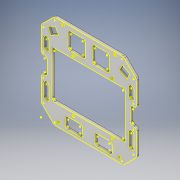
# Autodesk Inventor part: AnilloBaseVTOLv2
Saved by Autodesk Inventor 2019 (Build 230136000, 136)
## iProperties
Created: 2019-02-06
Part Number: AnilloBaseVTOLv2
Material: Generic
Document SubType Name: Modeling
Designer: Kenny
Density: 1 g/cm^3
Appearance: Default
Author: Kenny
Autodesk Inventor part; units mm, degrees
ref_plane "YZ Plane" through (0, 0, 0) normal (1, 0, 0) x (0, 1, 0)
ref_plane "XZ Plane" through (0, 0, 0) normal (0, 1, 0) x (-1, 0, 0)
ref_plane "XY Plane" through (0, 0, 0) normal (0, 0, 1) x (1, 0, 0)
sketch "Sketch1" plane through (0, 0, 0) normal (0, 0, 1) x (1, 0, 0)
  line L0 (0, 0) -> (110, 0)
  line L1 (110, 108) -> (0, 108)
  line L2 (55, 108) -> (55, 0) construction
  line L3 (12.5, 77) -> (97.5, 77)
  line L4 (97.5, 77) -> (97.5, 23)
  line L5 (97.5, 23) -> (12.5, 23)
  line L6 (12.5, 23) -> (12.5, 77)
  line L7 (-68.3542, 85.0055) -> (-13.3542, 85.0055) construction
  line L8 (-13.3542, 85.0055) -> (-13.3542, 15.0055) construction
  line L9 (-13.3542, 15.0055) -> (-68.3542, 15.0055) construction
  line L10 (-68.3542, 15.0055) -> (-68.3542, 85.0055) construction
  line L11 (49.5525, 105.4569) -> (59.7609, 105.4569) construction
  line L12 (59.7609, 105.4569) -> (59.7609, 101.2404) construction
  line L13 (59.7609, 101.2404) -> (49.5525, 101.2404) construction
  line L14 (49.5525, 101.2404) -> (49.5525, 105.4569) construction
  line L15 (0, 64) -> (7, 64)
  line L16 (7, 64) -> (7, 44)
  line L17 (7, 44) -> (0, 44)
  line L18 (0, 108) -> (0, 64)
  line L19 (0, 44) -> (0, 0)
  line L20 (110, 0) -> (110, 44)
  line L21 (110, 64) -> (110, 108)
  line L22 (59, 103) -> (79, 103)
  line L23 (79, 103) -> (79, 83)
  line L24 (79, 83) -> (59, 83)
  line L25 (59, 83) -> (59, 103)
  line L26 (31, 103) -> (51, 103)
  line L27 (51, 103) -> (51, 83)
  line L28 (51, 83) -> (31, 83)
  line L29 (31, 83) -> (31, 103)
  line L30 (3, 84) -> (9, 84)
  line L31 (9, 84) -> (9, 69)
  line L32 (9, 69) -> (3, 69)
  line L33 (3, 69) -> (3, 84)
  line L34 (101, 84) -> (107, 84)
  line L35 (107, 84) -> (107, 69)
  line L36 (107, 69) -> (101, 69)
  line L37 (101, 69) -> (101, 84)
  line L38 (62, 16) -> (82, 16)
  line L39 (82, 16) -> (82, 3)
  line L40 (82, 3) -> (62, 3)
  line L41 (62, 3) -> (62, 16)
  line L42 (28, 16) -> (48, 16)
  line L43 (48, 16) -> (48, 3)
  line L44 (48, 3) -> (28, 3)
  line L45 (28, 3) -> (28, 16)
  line L46 (110, 108) -> (110, 0) construction
  line L47 (110, 64) -> (103, 64)
  line L48 (103, 64) -> (103, 44)
  line L49 (103, 44) -> (110, 44)
  line L50 (9, 39) -> (3, 39)
  line L51 (3, 39) -> (3, 19)
  line L52 (3, 19) -> (9, 19)
  line L53 (9, 19) -> (9, 39)
  line L54 (101, 39) -> (107, 39)
  line L55 (107, 39) -> (107, 19)
  line L56 (107, 19) -> (101, 19)
  line L57 (101, 19) -> (101, 39)
  line L58 (0, 108) -> (20, 108)
  line L59 (20, 108) -> (20, 92) construction
  line L60 (20, 92) -> (0, 92) construction
  line L61 (0, 92) -> (0, 108)
  line L62 (110, 108) -> (90, 108)
  line L63 (90, 108) -> (90, 92) construction
  line L64 (90, 92) -> (110, 92) construction
  line L65 (110, 92) -> (110, 108)
  line L66 (90, 92) -> (98.9879, 87.6163)
  line L67 (98.9879, 87.6163) -> (102.4949, 94.8066)
  line L68 (102.4949, 94.8066) -> (93.507, 99.1904)
  line L69 (93.507, 99.1904) -> (90, 92)
  line L70 (20, 92) -> (11.0121, 87.6163)
  line L71 (11.0121, 87.6163) -> (7.5051, 94.8066)
  line L72 (7.5051, 94.8066) -> (16.493, 99.1904)
  line L73 (16.493, 99.1904) -> (20, 92)
  point P0 (25, 105)
  point P1 (85, 105)
  point P2 (20, 5)
  point P3 (90, 5)
  point P4 (-63.3542, 80.0055)
  point P5 (-63.3542, 20.0055)
  point P6 (-18.3542, 80.0055)
  point P7 (-18.3542, 20.0055)
  point P8 (37, 20)
  point P9 (82, 20)
  point P10 (37, 80)
  point P11 (82, 80)
  point P12 (104, 84)
  point P13 (6, 84)
  point P14 (41, 83)
  point P15 (72, 16)
  point P16 (6, 39)
  point P17 (104, 39)
  point P18 (41, 103)
  point P19 (69, 103)
  dimension "d0" = 60
  dimension "d1" = 100
  dimension "d2" = 70
  dimension "d3" = 110
  dimension "d4" = 108
  dimension "d6" = 35
  dimension "d7" = 5
  dimension "d8" = 85
  dimension "d9" = 54
  dimension "d11" = 45
  dimension "d12" = 60
  dimension "d14" = 23
  dimension "d15" = 55
  dimension "d16" = 70
  dimension "d17" = 5
  dimension "d18" = 5
  dimension "d23" = 28
  dimension "d24" = 20
  dimension "d29" = 7
  dimension "d30" = 20
  dimension "d35" = 12.5
  dimension "d36" = 12.5
  dimension "d38" = 20
  dimension "d39" = 20
  dimension "d40" = 25
  dimension "d41" = 45
  dimension "d42" = 28
  dimension "d43" = 20
  dimension "d44" = 20
  dimension "d46" = 31
  dimension "d47" = 6
  dimension "d48" = 15
  dimension "d49" = 6
  dimension "d50" = 15
  dimension "d51" = 3
  dimension "d52" = 3
  dimension "d53" = 31
  dimension "d54" = 20
  dimension "d55" = 13
  dimension "d56" = 20
  dimension "d57" = 13
  dimension "d58" = 28
  dimension "d59" = 28
  dimension "d60" = 7
  dimension "d62" = 7
  dimension "d63" = 20
  dimension "d64" = 6
  dimension "d65" = 20
  dimension "d66" = 6
  dimension "d67" = 20
  dimension "d68" = 3
  dimension "d69" = 3
  dimension "d70" = 5
  dimension "d71" = 5
  dimension "d72" = 5
  dimension "d73" = 7
  dimension "d74" = 19
  dimension "d75" = 5
  dimension "d137" = 20
  dimension "d138" = 16
  dimension "d139" = 20
  dimension "d140" = 16
  dimension "d203" = 10
  dimension "d204" = 8
  constraints: 140 end point, 32 parallel, 18 perpendicular, 15 horizontal, 10 midpoint, 9 horizontal alignment, 4 symmetric about line, 4 vertical alignment, 1 collinear, 2 other
  measures "d0" distance of point (85, 105) point (25, 105)
  measures "d1" vertical distance of point (90, 5) point (85, 105)
  measures "d2" distance of point (90, 5) point (20, 5)
  measures "d3" distance of L1.end L1.start
  measures "d4" distance of L1.start L0.end
  measures "d6" distance from line of L2 point (20, 5)
  measures "d7" distance from line of L0 point (20, 5)
  measures "d8" distance of L4.end L5.end
  measures "d9" distance of L3.end L4.end
  measures "d11" distance of point (-18.354, 80.005) point (-63.354, 80.005)
  measures "d12" distance of point (-63.354, 20.005) point (-63.354, 80.005)
  measures "d14" distance between parallel lines of L5 L0
  measures "d15" distance of L8.end L9.end
  measures "d16" distance of L7.end L8.end
  measures "d17" distance from line of L9 point (-18.354, 20.005)
  measures "d18" distance from line of L8 point (-18.354, 20.005)
  measures "d23" distance from line of L1 point (82, 80)
  measures "d24" distance from line of L0 point (37, 20)
  measures "d29" distance of L17.end L16.end
  measures "d30" distance of L15.end L16.end
  measures "d35" distance between parallel lines of L19 L6
  measures "d36" distance between parallel lines of L21 L4
  measures "d38" distance of L23.end L24.end
  measures "d39" distance of L22.end L23.end
  measures "d40" distance from line of L18 point (25, 105)
  measures "d41" distance of point (82, 80) point (37, 80)
  measures "d42" distance from line of L20 point (82, 20)
  measures "d43" distance of L27.end L28.end
  measures "d44" distance of L27.start L27.end
  measures "d46" distance between parallel lines of L18 L29
  measures "d47" distance of L31.end L32.end
  measures "d48" distance of L30.end L31.end
  measures "d49" distance of L35.end L37.start
  measures "d50" distance of L34.end L35.end
  measures "d51" distance between parallel lines of L33 L18
  measures "d52" distance between parallel lines of L21 L35
  measures "d53" distance between parallel lines of L21 L23
  measures "d54" distance of L39.end L40.end
  measures "d55" distance of L38.end L39.end
  measures "d56" distance of L43.end L44.end
  measures "d57" distance of L42.end L43.end
  measures "d58" distance between parallel lines of L20 L39
  measures "d59" distance between parallel lines of L19 L45
  measures "d60" distance between parallel lines of L42 L5
  measures "d62" distance of L21.start L47.end
  measures "d63" distance of L47.end L48.end
  measures "d64" distance of L52.end L51.end
  measures "d65" distance of L51.end L50.end
  measures "d66" distance of L55.end L56.end
  measures "d67" distance of L54.end L55.end
  measures "d68" distance between parallel lines of L46 L55
  measures "d69" distance between parallel lines of L19 L51
  measures "d70" distance between parallel lines of L15 L32
  measures "d71" distance between parallel lines of L50 L17
  measures "d72" distance between parallel lines of L26 L1
  measures "d73" distance between parallel lines of L38 L5
  measures "d74" distance between parallel lines of L0 L52
  measures "d75" distance between parallel lines of L54 L49
  measures "d137" distance of L59.end L60.end
  measures "d138" distance of L58.end L59.end
  measures "d139" distance of L64.start L64.end
  measures "d140" distance of L63.end L62.end
  measures "d203" distance of L67.end L68.end
  measures "d204" distance of L66.end L67.end
extrude "Extrusion1" add sketch "Sketch1" along normal blind 3
sketch "Holes" plane through (0, 0, 0) normal (0, 0, 1) x (1, 0, 0)
  line L0 (0, 0) -> (110, 0)
  line L1 (110, 108) -> (0, 108)
  line L2 (55, 108) -> (55, 0) construction
  line L3 (12.5, 77) -> (97.5, 77)
  line L4 (97.5, 77) -> (97.5, 23)
  line L5 (97.5, 23) -> (12.5, 23)
  line L6 (12.5, 23) -> (12.5, 77)
  line L7 (-68.3542, 85.0055) -> (-13.3542, 85.0055) construction
  line L8 (-13.3542, 85.0055) -> (-13.3542, 15.0055) construction
  line L9 (-13.3542, 15.0055) -> (-68.3542, 15.0055) construction
  line L10 (-68.3542, 15.0055) -> (-68.3542, 85.0055) construction
  line L11 (49.5525, 105.4569) -> (59.7609, 105.4569) construction
  line L12 (59.7609, 105.4569) -> (59.7609, 101.2404) construction
  line L13 (59.7609, 101.2404) -> (49.5525, 101.2404) construction
  line L14 (49.5525, 101.2404) -> (49.5525, 105.4569) construction
  line L15 (0, 64) -> (7, 64)
  line L16 (7, 64) -> (7, 44)
  line L17 (7, 44) -> (0, 44)
  line L18 (0, 108) -> (0, 64)
  line L19 (0, 44) -> (0, 0)
  line L20 (110, 0) -> (110, 44)
  line L21 (110, 64) -> (110, 108)
  line L22 (59, 103) -> (79, 103)
  line L23 (79, 103) -> (79, 83)
  line L24 (79, 83) -> (59, 83)
  line L25 (59, 83) -> (59, 103)
  line L26 (51, 103) -> (51, 83)
  line L27 (51, 83) -> (31, 83)
  line L28 (31, 103) -> (51, 103)
  line L29 (31, 83) -> (31, 103)
  line L30 (3, 89) -> (9, 89)
  line L31 (9, 89) -> (9, 69)
  line L32 (9, 69) -> (3, 69)
  line L33 (3, 69) -> (3, 89)
  line L34 (101, 89) -> (107, 89)
  line L35 (107, 89) -> (107, 69)
  line L36 (101, 69) -> (101, 89)
  line L37 (107, 69) -> (101, 69)
  line L38 (62, 16) -> (82, 16)
  line L39 (82, 16) -> (82, 3)
  line L40 (82, 3) -> (62, 3)
  line L41 (62, 3) -> (62, 16)
  line L42 (28, 16) -> (48, 16)
  line L43 (48, 16) -> (48, 3)
  line L44 (48, 3) -> (28, 3)
  line L45 (28, 3) -> (28, 16)
  line L46 (110, 108) -> (110, 0) construction
  line L47 (110, 64) -> (103, 64)
  line L48 (103, 64) -> (103, 44)
  line L49 (103, 44) -> (110, 44)
  line L50 (9, 39) -> (3, 39)
  line L51 (3, 39) -> (3, 19)
  line L52 (3, 19) -> (9, 19)
  line L53 (9, 19) -> (9, 39)
  line L54 (101, 39) -> (107, 39)
  line L55 (107, 39) -> (107, 19)
  line L56 (107, 19) -> (101, 19)
  line L57 (101, 19) -> (101, 39)
  line L58 (0, 108) -> (20, 108)
  line L59 (20, 108) -> (20, 92)
  line L60 (20, 92) -> (0, 92)
  line L61 (0, 92) -> (0, 108)
  line L62 (110, 108) -> (90, 108)
  line L63 (90, 108) -> (90, 92)
  line L64 (90, 92) -> (110, 92)
  line L65 (110, 92) -> (110, 108)
  point P0 (25, 105)
  point P1 (85, 105)
  point P2 (20, 5)
  point P3 (90, 5)
  point P4 (-63.3542, 80.0055)
  point P5 (-63.3542, 20.0055)
  point P6 (-18.3542, 80.0055)
  point P7 (-18.3542, 20.0055)
  point P8 (37, 20)
  point P9 (82, 20)
  point P10 (37, 80)
  point P11 (82, 80)
  point P12 (104, 89)
  point P13 (6, 89)
  point P14 (41, 83)
  point P15 (72, 16)
  point P16 (6, 39)
  point P17 (104, 39)
  point P18 (41, 103)
  point P19 (69, 103)
  dimension "d141" = 60
  dimension "d142" = 100
  dimension "d143" = 70
  dimension "d144" = 110
  dimension "d145" = 108
  dimension "d146" = 35
  dimension "d147" = 5
  dimension "d148" = 85
  dimension "d149" = 54
  dimension "d150" = 45
  dimension "d151" = 60
  dimension "d152" = 23
  dimension "d153" = 55
  dimension "d154" = 70
  dimension "d155" = 5
  dimension "d156" = 5
  dimension "d157" = 28
  dimension "d158" = 20
  dimension "d159" = 7
  dimension "d160" = 20
  dimension "d161" = 12.5
  dimension "d162" = 12.5
  dimension "d163" = 20
  dimension "d164" = 20
  dimension "d165" = 25
  dimension "d166" = 45
  dimension "d167" = 28
  dimension "d168" = 20
  dimension "d169" = 20
  dimension "d170" = 31
  dimension "d171" = 6
  dimension "d172" = 20
  dimension "d173" = 6
  dimension "d174" = 20
  dimension "d175" = 3
  dimension "d176" = 3
  dimension "d177" = 31
  dimension "d178" = 20
  dimension "d179" = 13
  dimension "d180" = 20
  dimension "d181" = 13
  dimension "d182" = 28
  dimension "d183" = 28
  dimension "d184" = 7
  dimension "d185" = 7
  dimension "d186" = 20
  dimension "d187" = 6
  dimension "d188" = 20
  dimension "d189" = 6
  dimension "d190" = 20
  dimension "d191" = 3
  dimension "d192" = 3
  dimension "d193" = 5
  dimension "d194" = 5
  dimension "d195" = 5
  dimension "d196" = 7
  dimension "d197" = 19
  dimension "d198" = 5
  dimension "d199" = 20
  dimension "d200" = 16
  dimension "d201" = 20
  dimension "d202" = 16
  constraints: 124 end point, 30 parallel, 17 perpendicular, 15 horizontal, 10 midpoint, 9 horizontal alignment, 4 vertical alignment, 1 collinear, 2 other
  measures "d141" distance of point (85, 105) point (25, 105)
  measures "d142" vertical distance of point (90, 5) point (85, 105)
  measures "d143" distance of point (90, 5) point (20, 5)
  measures "d144" distance of L1.end L1.start
  measures "d145" distance of L1.start L0.end
  measures "d146" distance from line of L2 point (20, 5)
  measures "d147" distance from line of L0 point (20, 5)
  measures "d148" distance of L4.end L5.end
  measures "d149" distance of L3.end L4.end
  measures "d150" distance of point (-18.354, 80.005) point (-63.354, 80.005)
  measures "d151" distance of point (-63.354, 20.005) point (-63.354, 80.005)
  measures "d152" distance between parallel lines of L5 L0
  measures "d153" distance of L8.end L9.end
  measures "d154" distance of L7.end L8.end
  measures "d155" distance from line of L9 point (-18.354, 20.005)
  measures "d156" distance from line of L8 point (-18.354, 20.005)
  measures "d157" distance from line of L1 point (82, 80)
  measures "d158" distance from line of L0 point (37, 20)
  measures "d159" distance of L17.end L16.end
  measures "d160" distance of L15.end L16.end
  measures "d161" distance between parallel lines of L19 L6
  measures "d162" distance between parallel lines of L21 L4
  measures "d163" distance of L23.end L24.end
  measures "d164" distance of L22.end L23.end
  measures "d165" distance from line of L18 point (25, 105)
  measures "d166" distance of point (82, 80) point (37, 80)
  measures "d167" distance from line of L20 point (82, 20)
  measures "d168" distance of L26.end L27.end
  measures "d169" distance of L26.start L26.end
  measures "d170" distance between parallel lines of L18 L29
  measures "d171" distance of L31.end L32.end
  measures "d172" distance of L30.end L31.end
  measures "d173" distance of L35.end L36.start
  measures "d174" distance of L34.end L35.end
  measures "d175" distance between parallel lines of L33 L18
  measures "d176" distance between parallel lines of L21 L35
  measures "d177" distance between parallel lines of L21 L23
  measures "d178" distance of L39.end L40.end
  measures "d179" distance of L38.end L39.end
  measures "d180" distance of L43.end L44.end
  measures "d181" distance of L42.end L43.end
  measures "d182" distance between parallel lines of L20 L39
  measures "d183" distance between parallel lines of L19 L45
  measures "d184" distance between parallel lines of L42 L5
  measures "d185" distance of L21.start L47.end
  measures "d186" distance of L47.end L48.end
  measures "d187" distance of L52.end L51.end
  measures "d188" distance of L51.end L50.end
  measures "d189" distance of L55.end L56.end
  measures "d190" distance of L54.end L55.end
  measures "d191" distance between parallel lines of L46 L55
  measures "d192" distance between parallel lines of L19 L51
  measures "d193" distance between parallel lines of L15 L32
  measures "d194" distance between parallel lines of L50 L17
  measures "d195" distance between parallel lines of L28 L1
  measures "d196" distance between parallel lines of L38 L5
  measures "d197" distance between parallel lines of L0 L52
  measures "d198" distance between parallel lines of L54 L49
  measures "d199" distance of L59.end L60.end
  measures "d200" distance of L58.end L59.end
  measures "d201" distance of L64.end L63.end
  measures "d202" distance of L63.end L62.end
hole "Hole1" at (25, 105, 0) at (85, 105, 0) at (20, 5, 0) at (90, 5, 0) at (-63.3542, 80.0055, 0) at (-63.3542, 20.0055, 0) at (-18.3542, 80.0055, 0) at (-18.3542, 20.0055, 0) at (37, 20, 0) at (82, 20, 0) at (37, 80, 0) at (82, 80, 0) direction (0, 0, 1) diameter 3.3 end through all
fillet "Fillet1" radius 3 44 edges at (31, 83, 1.5) (31, 103, 1.5) (51, 103, 1.5) (51, 83, 1.5) (59, 83, 1.5) (59, 103, 1.5) (79, 103, 1.5) (79, 83, 1.5) (101, 84, 1.5) (107, 84, 1.5) (107, 69, 1.5) (101, 69, 1.5) (103, 64, 1.5) (110, 64, 1.5) (110, 44, 1.5) (103, 44, 1.5) (101, 39, 1.5) (107, 39, 1.5) (107, 19, 1.5) (101, 19, 1.5) (82, 3, 1.5) (82, 16, 1.5) (62, 16, 1.5) (62, 3, 1.5) (48, 3, 1.5) (48, 16, 1.5) (28, 16, 1.5) (28, 3, 1.5) (9, 19, 1.5) (3, 19, 1.5) (9, 39, 1.5) (3, 39, 1.5) (7, 44, 1.5) (7, 64, 1.5) (0, 64, 1.5) (0, 44, 1.5) (3, 69, 1.5) (3, 84, 1.5) (9, 84, 1.5) (9, 69, 1.5) (12.5, 23, 1.5) (12.5, 77, 1.5) (97.5, 77, 1.5) (97.5, 23, 1.5)
chamfer "Chamfer1" distance 15 angle 45 4 edges at (110, 108, 1.5) (0, 108, 1.5) (110, 0, 1.5) (0, 0, 1.5)
fillet "Fillet2" radius 3 8 edges at (95, 108, 1.5) (110, 93, 1.5) (110, 15, 1.5) (15, 108, 1.5) (0, 93, 1.5) (0, 15, 1.5) (95, 0, 1.5) (15, 0, 1.5)
sketch "Sketch5" plane through (0, 0, 3) normal (0, 0, 1) x (1, 0, 0)
  circle A0 centre (37, 80) radius 1.65 projected
  circle A1 centre (37, 20) radius 1.65 projected
  circle A2 centre (20, 5) radius 1.65 projected
  circle A3 centre (25, 105) radius 1.65 projected
  circle A4 centre (85, 105) radius 1.65 projected
  circle A5 centre (90, 5) radius 1.65 projected
  circle A6 centre (82, 20) radius 1.65 projected
  circle A7 centre (82, 80) radius 1.65 projected
  line L0 (97.5, 74) -> (97.5, 26) projected
  arc A8 (94.5, 23) -> (97.5, 26) centre (94.5, 26) ccw projected
  line L1 (94.5, 23) -> (15.5, 23) projected
  arc A9 (12.5, 26) -> (15.5, 23) centre (15.5, 26) ccw projected
  line L2 (12.5, 26) -> (12.5, 74) projected
  arc A10 (15.5, 77) -> (12.5, 74) centre (15.5, 74) ccw projected
  line L3 (15.5, 77) -> (94.5, 77) projected
  arc A11 (97.5, 74) -> (94.5, 77) centre (94.5, 74) ccw projected
  line L4 (48, 83) -> (34, 83) projected
  arc A12 (31, 86) -> (34, 83) centre (34, 86) ccw projected
  line L5 (31, 86) -> (31, 100) projected
  arc A13 (34, 103) -> (31, 100) centre (34, 100) ccw projected
  line L6 (34, 103) -> (48, 103) projected
  arc A14 (51, 100) -> (48, 103) centre (48, 100) ccw projected
  line L7 (51, 100) -> (51, 86) projected
  arc A15 (48, 83) -> (51, 86) centre (48, 86) ccw projected
  line L8 (79, 100) -> (79, 86) projected
  arc A16 (76, 83) -> (79, 86) centre (76, 86) ccw projected
  line L9 (76, 83) -> (62, 83) projected
  arc A17 (59, 86) -> (62, 83) centre (62, 86) ccw projected
  line L10 (59, 86) -> (59, 100) projected
  arc A18 (62, 103) -> (59, 100) centre (62, 100) ccw projected
  line L11 (62, 103) -> (76, 103) projected
  arc A19 (79, 100) -> (76, 103) centre (76, 100) ccw projected
  line L12 (48, 13) -> (48, 6) projected
  arc A20 (45, 3) -> (48, 6) centre (45, 6) ccw projected
  line L13 (45, 3) -> (31, 3) projected
  arc A21 (28, 6) -> (31, 3) centre (31, 6) ccw projected
  line L14 (28, 6) -> (28, 13) projected
  arc A22 (31, 16) -> (28, 13) centre (31, 13) ccw projected
  line L15 (31, 16) -> (45, 16) projected
  arc A23 (48, 13) -> (45, 16) centre (45, 13) ccw projected
  line L16 (82, 13) -> (82, 6) projected
  arc A24 (79, 3) -> (82, 6) centre (79, 6) ccw projected
  line L17 (79, 3) -> (65, 3) projected
  arc A25 (62, 6) -> (65, 3) centre (65, 6) ccw projected
  line L18 (62, 6) -> (62, 13) projected
  arc A26 (65, 16) -> (62, 13) centre (65, 13) ccw projected
  line L19 (65, 16) -> (79, 16) projected
  arc A27 (82, 13) -> (79, 16) centre (79, 13) ccw projected
  line L20 (107, 36) -> (107, 22) projected
  arc A28 (101, 22) -> (107, 22) centre (104, 22) ccw projected
  line L21 (101, 22) -> (101, 36) projected
  arc A29 (107, 36) -> (101, 36) centre (104, 36) ccw projected
  line L22 (9, 36) -> (9, 22) projected
  arc A30 (3, 22) -> (9, 22) centre (6, 22) ccw projected
  line L23 (3, 22) -> (3, 36) projected
  arc A31 (9, 36) -> (3, 36) centre (6, 36) ccw projected
  line L24 (107, 81) -> (107, 72) projected
  arc A32 (101, 72) -> (107, 72) centre (104, 72) ccw projected
  line L25 (101, 72) -> (101, 81) projected
  arc A33 (107, 81) -> (101, 81) centre (104, 81) ccw projected
  line L26 (9, 81) -> (9, 72) projected
  arc A34 (3, 72) -> (9, 72) centre (6, 72) ccw projected
  line L27 (3, 72) -> (3, 81) projected
  arc A35 (9, 81) -> (3, 81) centre (6, 81) ccw projected
  line L28 (11.0121, 87.6163) -> (7.5051, 94.8066) projected
  line L29 (7.5051, 94.8066) -> (16.493, 99.1904) projected
  line L30 (16.493, 99.1904) -> (20, 92) projected
  line L31 (20, 92) -> (11.0121, 87.6163) projected
  line L32 (90, 92) -> (93.507, 99.1904) projected
  line L33 (93.507, 99.1904) -> (102.4949, 94.8066) projected
  line L34 (102.4949, 94.8066) -> (98.9879, 87.6163) projected
  line L35 (98.9879, 87.6163) -> (90, 92) projected
  arc A36 (14.1213, 0.8787) -> (16.2426, 0) centre (16.2426, 3) ccw projected
  line L36 (16.2426, 0) -> (93.7574, 0) projected
  arc A37 (93.7574, 0) -> (95.8787, 0.8787) centre (93.7574, 3) ccw projected
  line L37 (109.1213, 14.1213) -> (95.8787, 0.8787) projected
  arc A38 (109.1213, 14.1213) -> (110, 16.2426) centre (107, 16.2426) ccw projected
  line L38 (110, 16.2426) -> (110, 41) projected
  arc A39 (110, 41) -> (107, 44) centre (107, 41) ccw projected
  line L39 (107, 44) -> (106, 44) projected
  arc A40 (103, 47) -> (106, 44) centre (106, 47) ccw projected
  line L40 (103, 47) -> (103, 61) projected
  arc A41 (106, 64) -> (103, 61) centre (106, 61) ccw projected
  line L41 (106, 64) -> (107, 64) projected
  arc A42 (107, 64) -> (110, 67) centre (107, 67) ccw projected
  line L42 (110, 67) -> (110, 91.7574) projected
  arc A43 (110, 91.7574) -> (109.1213, 93.8787) centre (107, 91.7574) ccw projected
  line L43 (95.8787, 107.1213) -> (109.1213, 93.8787) projected
  arc A44 (95.8787, 107.1213) -> (93.7574, 108) centre (93.7574, 105) ccw projected
  line L44 (93.7574, 108) -> (16.2426, 108) projected
  arc A45 (16.2426, 108) -> (14.1213, 107.1213) centre (16.2426, 105) ccw projected
  line L45 (0.8787, 93.8787) -> (14.1213, 107.1213) projected
  arc A46 (0.8787, 93.8787) -> (0, 91.7574) centre (3, 91.7574) ccw projected
  line L46 (0, 91.7574) -> (0, 67) projected
  arc A47 (0, 67) -> (3, 64) centre (3, 67) ccw projected
  line L47 (3, 64) -> (4, 64) projected
  arc A48 (7, 61) -> (4, 64) centre (4, 61) ccw projected
  line L48 (7, 61) -> (7, 47) projected
  arc A49 (4, 44) -> (7, 47) centre (4, 47) ccw projected
  line L49 (4, 44) -> (3, 44) projected
  arc A50 (3, 44) -> (0, 41) centre (3, 41) ccw projected
  line L50 (0, 41) -> (0, 16.2426) projected
  arc A51 (0, 16.2426) -> (0.8787, 14.1213) centre (3, 16.2426) ccw projected
  line L51 (14.1213, 0.8787) -> (0.8787, 14.1213) projected
  point P0 (0, 0)
body "Solid1"
